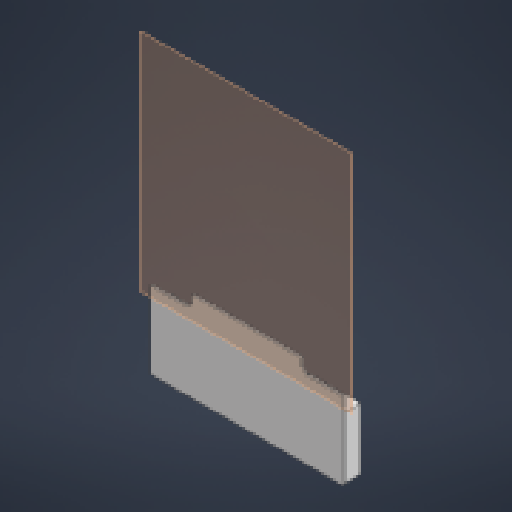
# Autodesk Inventor part: Part2
Saved by Autodesk Inventor 2026.3 (Build 303398000, 398)
## iProperties
Created: 2026-07-07
Part Number: Part2
Material: Generic
Document SubType Name: Modeling
Designer: user
Density: 1 g/cm^3
Appearance: Default
Author: user
Autodesk Inventor part; units mm, degrees
ref_plane "YZ Plane" through (0, 0, 0) normal (1, 0, 0) x (0, 1, 0)
ref_plane "XZ Plane" through (0, 0, 0) normal (0, 1, 0) x (-1, 0, 0)
ref_plane "XY Plane" through (0, 0, 0) normal (0, 0, 1) x (1, 0, 0)
ref_plane "Work Plane1" through (0, 0, 0) normal (0, 0, 1) x (1, 0, 0)
sketch "Sketch1" plane through (0, 0, 0) normal (0, 0, 1) x (1, 0, 0)
  line L0 (93, -160) -> (85, -152) projected
  line L1 (150, -160) -> (93, -160) projected
  line L2 (150, -27.5) -> (150, -160) projected
  line L3 (110, -27.5) -> (150, -27.5) projected
  line L4 (110, 47.5) -> (110, -27.5) projected
  line L5 (150, 47.5) -> (110, 47.5) projected
  line L6 (150, 160) -> (150, 47.5) projected
  line L7 (-150, 160) -> (150, 160) projected
  line L8 (-150, 47.5) -> (-150, 160) projected
  line L9 (-110, 47.5) -> (-150, 47.5) projected
  line L10 (-110, -27.5) -> (-110, 47.5) projected
  line L11 (-150, -27.5) -> (-110, -27.5) projected
  line L12 (-150, -160) -> (-150, -27.5) projected
  line L13 (-93, -160) -> (-150, -160) projected
  line L14 (-85, -152) -> (-93, -160) projected
  line L15 (-85, -140) -> (-85, -152) projected
  line L16 (85, -140) -> (-85, -140) projected
  line L17 (85, -152) -> (85, -140) projected
  line L18 (-150, -280.0045) -> (150, -280.0045)
  line L19 (150, -280.0045) -> (150, -118.8161)
  line L20 (150, -118.8161) -> (-150, -118.8161)
  line L21 (-150, -118.8161) -> (-150, -280.0045)
  point P0 (0, 0)
  constraints: 8 end point, 2 parallel, 1 horizontal, 1 perpendicular, 1 point on line
extrude "Extrusion1" add sketch "Sketch1" against normal blind 3 contours L1 L19 L18 L21 L13 L14 L15 L16 L17 L0
sketch "Sketch2" plane through (0, 0, -3) normal (0, 0, -1) x (-1, 0, 0)
  line L0 (-149, -279.3573) -> (-149, -162.5589) projected
  line L1 (-79, -279.1787) -> (-149, -279.1787) projected
  line L2 (-149, -279.1787) -> (147.9655, -279.1787)
  line L3 (147.9655, -279.1787) -> (147.9655, -183.5488)
  line L4 (147.9655, -183.5488) -> (-149, -183.5488)
  line L5 (-149, -183.5488) -> (-149, -279.1787)
  point P0 (0, 0)
  point P1 (-149, -183.5488)
  constraints: 8 end point, 2 parallel, 1 horizontal, 1 perpendicular
extrude "Extrusion2" add sketch "Sketch2" along normal blind 25.4
sketch "Sketch3" plane through (0, 0, -28.4) normal (0, 0, -1) x (-1, 0, 0)
  line L0 (75.5, -193.4434) -> (-74.5, -193.4434) projected
  line L1 (-74.5, -193.4434) -> (-74.5, -316.9258) projected
  line L2 (-74.5, -316.9258) -> (75.5, -316.9258) projected
  line L3 (75.5, -316.9258) -> (75.5, -193.4434) projected
  line L4 (63.5, -304.9759) -> (-62.5, -304.9759) projected
  line L5 (-62.5, -304.9759) -> (-62.5, -205.3933) projected
  line L6 (-62.5, -205.3933) -> (63.5, -205.3933) projected
  line L7 (63.5, -205.3933) -> (63.5, -304.9759) projected
  line L8 (-78.5724, -320.9982) -> (-78.5724, -189.371)
  line L9 (-78.5724, -189.371) -> (79.5724, -189.371)
  line L10 (79.5724, -189.371) -> (79.5724, -320.9982)
  line L11 (79.5724, -320.9982) -> (-78.5724, -320.9982)
  point P0 (0, 0)
  constraints: 8 end point, 3 other
extrude "Extrusion3" cut sketch "Sketch3" against normal blind 50.8 contours L3 L2 L1 L0 | L4 L5 L6 L7 | L8 L9 L10 L11
body "Solid1"
